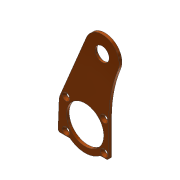
# Autodesk Inventor part: UPPER_LEG_MIDDLE_FRAME_3
Saved by Autodesk Inventor 2019.4 (Build 234330000, 330)
## iProperties
Created: 2019-11-14
Part Number: UPPER_LEG_MIDDLE_FRAME_3
Material: 一般
Document SubType Name: Modeling
Designer: y6tada
Density: 1 g/cm^3
Appearance: 滑らか - 淡いオレンジ
Author: y6tada
Autodesk Inventor part; units mm, degrees
ref_plane "YZ Plane" through (0, 0, 0) normal (1, 0, 0) x (0, 1, 0)
ref_plane "XZ Plane" through (0, 0, 0) normal (0, 1, 0) x (-1, 0, 0)
ref_plane "XY Plane" through (0, 0, 0) normal (0, 0, 1) x (1, 0, 0)
sketch "スケッチ1" plane through (0, 0, 0) normal (0, 0, 1) x (1, 0, 0)
  circle A0 centre (0, 15.5) radius 1.5 construction
  circle A1 centre (-13.5, 26) radius 1.25 construction
  circle A2 centre (13.5, 26) radius 1.25 construction
  circle A3 centre (-13.5, 5) radius 1.25 construction
  circle A4 centre (13.5, 5) radius 1.25 construction
  arc A5 (23.2244, 60.3803) -> (0.9204, 69.5092) centre (12.061, 64.9168) ccw
  line L0 (0.9204, 69.5092) -> (-16.5047, 27.2386)
  arc A6 (23.2244, 60.3803) -> (16.75, 27.25) centre (104.7526, 27.25) ccw
  arc A7 (-16.5047, 27.2386) -> (-16.75, 26) centre (-13.5, 26) ccw
  circle A8 centre (0, 15.5) radius 13.25
  line L1 (-16.75, 26) -> (-16.75, 3)
  line L2 (-15.75, 2) -> (-11.4155, 2)
  line L3 (11.4155, 2) -> (15.75, 2)
  arc A9 (-10.2294, 1.6104) -> (10.2294, 1.6104) centre (0, 15.5) ccw
  line L4 (16.75, 27.25) -> (16.75, 3)
  line L5 (15.75, 2) -> (16.75, 3)
  line L6 (-15.75, 2) -> (-16.75, 3)
  arc A10 (-10.2294, 1.6104) -> (-11.4155, 2) centre (-11.4155, 0) ccw
  arc A11 (11.4155, 2) -> (10.2294, 1.6104) centre (11.4155, 0) ccw
  circle A12 centre (12.061, 64.9168) radius 5 construction
  line L7 (0, 15.5) -> (0, 44.2694) construction
  point P0 (0, 0)
  point P1 (-10.7384, 2)
  point P2 (10.7384, 2)
  point P3 (16.75, 2)
  point P4 (-16.75, 2)
  dimension "d0" = 26.5
  dimension "d1" = 4
  dimension "d2" = 3
  dimension "d3" = 1
  dimension "d4" = 1
  dimension "d5" = 1
  dimension "d6" = 1
  dimension "d7" = 2
  dimension "d27" = 12.05
  constraints: 16 end point, 14 point on circle, 9 tangent, 8 centre point, 6 point on line, 3 concentric, 3 vertical, 2 coincident, 2 horizontal, 1 collinear, 1 equal radius, 3 other
  measures "d0" diameter of A8
  measures "d1" radial gap between concentric circles of A8 A9
  measures "d2" distance from line of L2 A3.centre
  measures "d3" distance of L3.end point (16.75, 2)
  measures "d4" distance of L4.end point (16.75, 2)
  measures "d5" distance of L2.start point (-16.75, 2)
  measures "d6" distance of L1.end point (-16.75, 2)
  measures "d7" radius of A10
  measures "d27" radius of A5
extrude "押し出し1" add sketch "スケッチ1" along normal blind 2
hole "穴1" at (12.061, 64.9168, 0) direction (0, 0, 1) diameter 10 end through all counterbore diameter 11.3 counterbore depth 0.65
sketch "スケッチ2" plane through (0, 0, 2) normal (0, 0, 1) x (1, 0, 0)
  circle A0 centre (13.5, 5) radius 1.25 construction
  circle A1 centre (-13.5, 5) radius 1.25 construction
  circle A2 centre (-13.5, 26) radius 1.25 construction
  circle A3 centre (13.5, 26) radius 1.25 construction
  point P0 (0, 0)
  constraints: 4 coincident
hole "穴2" at (-13.5, 5, 2) at (-13.5, 26, 2) at (13.5, 26, 2) at (13.5, 5, 2) direction (0, 0, -1) diameter 2.5 end through all countersink diameter 5.4 countersink angle 90
equation "\"d4\" = d3"
equation "\"d5\" = d3"
equation "\"d6\" = d5"
